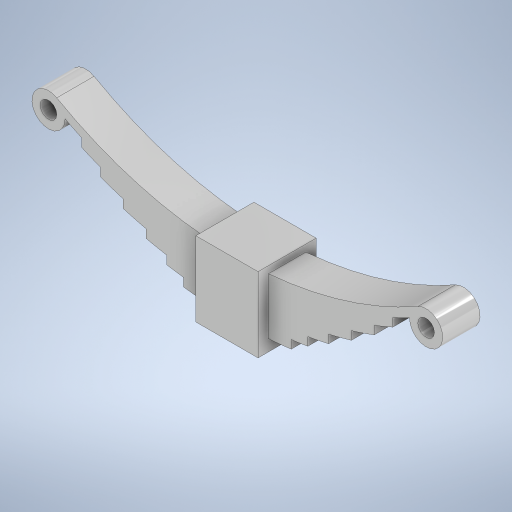
# Autodesk Inventor part: HUDSON-1-09-LEAF SPRING PACK
Saved by Autodesk Inventor 2024.2 (Build 282272000, 272)
## iProperties
Created: 2024-10-08
Part Number: HUDSON-1-09-LEAF SPRING PACK
Material: Generic
Document SubType Name: Modeling
Designer: Jimena Brenes
Density: 1 g/cm^3
Appearance: Aluminum - Polished
Author: Jimena Brenes
Autodesk Inventor part; units mm, degrees
ref_plane "YZ Plane" through (0, 0, 0) normal (1, 0, 0) x (0, 1, 0)
ref_plane "XZ Plane" through (0, 0, 0) normal (0, 1, 0) x (-1, 0, 0)
ref_plane "XY Plane" through (0, 0, 0) normal (0, 0, 1) x (1, 0, 0)
sketch "Sketch1" plane through (0, 0, 0) normal (0, 0, 1) x (1, 0, 0)
  arc A0 (1.9783, 3.4766) -> (3.9987, 0.1008) centre (0, 0) ccw
  arc A1 (87.0013, 0.1008) -> (89.0217, 3.4766) centre (91, 0) ccw
  line L0 (0, 0) -> (109, 0) construction
  line L1 (8, -1.8544) -> (8, -3.8544)
  line L2 (83, -1.8544) -> (83, -3.8544)
  line L3 (45.5, 0) -> (45.5, -69) construction
  line L4 (12.5, -5.7261) -> (12.5, -7.7261)
  line L5 (78.5, -5.7261) -> (78.5, -7.7261)
  line L6 (18, -9.6033) -> (18, -11.6033)
  line L7 (73, -9.6033) -> (73, -11.6033)
  line L8 (23.5, -13.0781) -> (23.5, -15.0781)
  line L9 (67.5, -13.0781) -> (67.5, -15.0781)
  line L10 (28.5, -16.0985) -> (28.5, -18.0985)
  line L11 (62.5, -16.0985) -> (62.5, -18.0985)
  line L12 (32.5, -18.7085) -> (32.5, -20.7085)
  line L13 (58.5, -18.7085) -> (58.5, -20.7085)
  circle A2 centre (91, 0) radius 2
  circle A3 centre (0, 0) radius 2
  line L14 (38, -6.0391) -> (53, -6.0391)
  line L15 (53, -6.0391) -> (53, -24.0391)
  line L16 (53, -24.0391) -> (38, -24.0391)
  line L17 (38, -24.0391) -> (38, -6.0391)
  arc A4 (3.9987, 0.1008) -> (38, -9.726) centre (45.5, 79.9609) ccw
  arc A5 (53, -9.726) -> (87.0013, 0.1008) centre (45.5, 79.9609) ccw
  line L18 (0, -8.0391) -> (38, -8.0391) construction
  line L19 (53, -8.0391) -> (95.0831, -8.0391) construction
  arc A6 (1.9783, 3.4766) -> (38, -7.7189) centre (45.5, 79.9609) ccw
  arc A7 (53, -7.7189) -> (89.0217, 3.4766) centre (45.5, 79.9609) ccw
  arc A8 (8, -3.8544) -> (38, -11.5542) centre (45.5, 79.9609) ccw
  arc A9 (53, -11.5542) -> (83, -3.8544) centre (45.5, 79.9609) ccw
  arc A10 (12.5, -7.7261) -> (38, -13.4294) centre (45.5, 79.9609) ccw
  arc A11 (53, -13.4294) -> (78.5, -7.7261) centre (45.5, 79.9609) ccw
  arc A12 (18, -11.6033) -> (38, -15.3492) centre (45.5, 79.9609) ccw
  arc A13 (53, -15.3492) -> (73, -11.6033) centre (45.5, 79.9609) ccw
  arc A14 (23.5, -15.0781) -> (38, -17.3025) centre (45.5, 79.9609) ccw
  arc A15 (53, -17.3025) -> (67.5, -15.0781) centre (45.5, 79.9609) ccw
  arc A16 (28.5, -18.0985) -> (38, -19.2782) centre (45.5, 79.9609) ccw
  arc A17 (53, -19.2782) -> (62.5, -18.0985) centre (45.5, 79.9609) ccw
  arc A18 (32.5, -20.7085) -> (38, -21.267) centre (45.5, 79.9609) ccw
  arc A19 (53, -21.267) -> (58.5, -20.7085) centre (45.5, 79.9609) ccw
  dimension "d53" = 15
  dimension "d1" = 8
  dimension "d2" = 91
  dimension "d10" = 2
  dimension "d11" = 2
  dimension "d13" = 45.5
  dimension "d16" = 2
  dimension "d17" = 2
  dimension "d19" = 33
  dimension "d20" = 37.5
  dimension "d21" = 2
  dimension "d22" = 2
  dimension "d23" = 27.5
  dimension "d24" = 27.5
  dimension "d25" = 2
  dimension "d26" = 2
  dimension "d27" = 22
  dimension "d29" = 2
  dimension "d30" = 2
  dimension "d32" = 17
  dimension "d33" = 2
  dimension "d34" = 2
  dimension "d35" = 13
  dimension "d37" = 4
  dimension "d38" = 4
  dimension "d52" = 18
  dimension "d54" = 7.5
  constraints: 48 point on circle, 36 end point, 20 centre point, 13 vertical, 10 coincident, 5 horizontal, 2 point on line, 2 tangent, 1 parallel, 24 other
  measures "d1" diameter of A1
  measures "d2" distance of A1.centre point (0, 0)
  measures "d10" distance of L1.end L1.start
  measures "d11" distance of L2.start L2.end
  measures "d13" distance from line of point (0, 0) L3
  measures "d16" distance of L4.end L4.start
  measures "d17" distance of L5.start L5.end
  measures "d19" distance between parallel lines of L3 L5
  measures "d20" distance between parallel lines of L3 L1
  measures "d21" distance of L6.start L6.end
  measures "d22" distance of L7.start L7.end
  measures "d23" distance between parallel lines of L3 L7
  measures "d24" distance between parallel lines of L3 L6
  measures "d25" distance of L8.start L8.end
  measures "d26" distance of L9.end L9.start
  measures "d27" distance between parallel lines of L3 L8
  measures "d29" distance of L10.end L10.start
  measures "d30" distance of L11.start L11.end
  measures "d32" distance between parallel lines of L3 L10
  measures "d33" distance of L12.start L12.end
  measures "d34" distance of L13.end L13.start
  measures "d35" distance between parallel lines of L3 L12
  measures "d37" diameter of A2
  measures "d38" diameter of A3
  measures "d52" distance between parallel lines of L16 L14
extrude "Extrusion5" add sketch "Sketch1" along normal mid plane 14 contours L17 L14 L15 L16
extrude "Extrusion6" add sketch "Sketch1" along normal mid plane 9 contours A6 L17 A4 A0 | A4 L17 A8 L1 | L17 A10 L4 A8 | L17 A12 L6 A10 | A7 A1 A5 L15 | L17 A14 L8 A12 | A5 L2 A9 L15 | L17 A16 L10 A14 | A9 L5 A11 L15 | L17 A18 L12 A16 | A11 L7 A13 L15 | A13 L9 A15 L15 | A15 L11 A17 L15 | A17 L13 A19 L15
sketch "Sketch2" plane through (38, -24.0391, 7) normal (0, -1, 0) x (1, 0, 0)
  circle A0 centre (7.5, -7) radius 4
  line L0 (15, -14) -> (0, -14) projected
  line L1 (0, -14) -> (0, 0) projected
  point P0 (-38, -7)
  dimension "d59" = 8
  dimension "d60" = 7
  dimension "d61" = 7.5
  constraints: 1 centre point
  measures "d59" diameter of A0
  measures "d60" distance from line of L0 A0.centre
  measures "d61" distance from line of L1 A0.centre
hole "Hole1" at (45.5, -24.0391, 0) direction (0, 1, 0) diameter 8 depth 11.72
equation "\"d19\" = d18"
equation "\"d32\" = d31"
equation "\"d18\" = 33"
equation "\"d31\" = 17"
body "Solid1"
